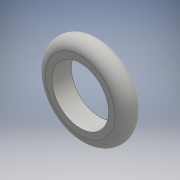
# Autodesk Inventor part: wheel1
Saved by Autodesk Inventor 2016 (Build 200138000, 138)
## iProperties
Created: 2016-01-30
Part Number: wheel1
Material: Generic
Document SubType Name: Modeling
Designer: Carlo
Density: 1 g/cm^3
Appearance: Default
Author: Carlo
Autodesk Inventor part; units mm, degrees
ref_plane "YZ Plane" through (0, 0, 0) normal (1, 0, 0) x (0, 1, 0)
ref_plane "XZ Plane" through (0, 0, 0) normal (0, 1, 0) x (-1, 0, 0)
ref_plane "XY Plane" through (0, 0, 0) normal (0, 0, 1) x (1, 0, 0)
sketch "Sketch1" plane through (0, 0, 0) normal (0, 1, 0) x (-1, 0, 0)
  circle A0 centre (0, 0) radius 55
  circle A1 centre (0, 0) radius 35
  dimension "d0" = 110
  dimension "d1" = 70
  constraints: 2 centre point, 2 coincident
  measures "d0" diameter of A0
  measures "d1" diameter of A1
extrude "Extrusion1" add sketch "Sketch1" along normal blind 24
fillet "Fillet1" radius 12 2 edges at (55, 24, 0) (55, 0, 0)
body "Solid1"
